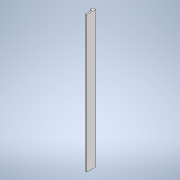
# Autodesk Inventor part: UgolUkrep
Saved by Autodesk Inventor 2022 (Build 260153000, 153)
## iProperties
Created: 2023-08-15
Part Number: UgolUkrep
Material: Generic
Document SubType Name: Modeling
Designer: Kippi
Density: 1 g/cm^3
Appearance: Default
Author: Kippi
Autodesk Inventor part; units mm, degrees
ref_plane "YZ Plane" through (0, 0, 0) normal (1, 0, 0) x (0, 1, 0)
ref_plane "XZ Plane" through (0, 0, 0) normal (0, 1, 0) x (-1, 0, 0)
ref_plane "XY Plane" through (0, 0, 0) normal (0, 0, 1) x (1, 0, 0)
sketch "Sketch1" plane through (0, 0, 0) normal (0, 1, 0) x (-1, 0, 0)
  point P0 (0, 0)
sketch "Sketch2" plane through (0, 0, 0) normal (0, 1, 0) x (-1, 0, 0)
  line L0 (3.7143, 31.4286) -> (-6.2857, 31.4286)
  line L1 (-6.2857, 31.4286) -> (-6.2857, -33.5714)
  line L2 (-6.2857, -33.5714) -> (3.7143, -33.5714)
  line L3 (3.7143, -33.5714) -> (3.7143, 31.4286)
  line L4 (13.7143, -12.5714) -> (3.7143, -12.5714)
  line L5 (3.7143, -12.5714) -> (3.7143, -33.5714)
  line L6 (3.7143, -33.5714) -> (13.7143, -33.5714)
  line L7 (13.7143, -33.5714) -> (13.7143, -12.5714)
  point P0 (0, 0)
  dimension "d0" = 44
  dimension "d1" = 10
  dimension "d2" = 10
  dimension "d3" = 65
  constraints: 16 end point, 4 parallel, 2 horizontal, 2 perpendicular
  measures "d0" distance between parallel lines of L0 L4
  measures "d1" distance of L0.start L0.end
  measures "d2" distance of L4.start L4.end
  measures "d3" distance of L0.end L1.end
extrude "Extrusion1" add sketch "Sketch2" along normal blind 1000
body "Solid1"
